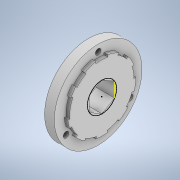
# Autodesk Inventor part: wheel_gearing_mount_short
Saved by Autodesk Inventor 2021 (Build 250183000, 183)
## iProperties
Created: 2021-01-10
Part Number: wheel_gearing_mount_short
Material: Generic
Document SubType Name: Modeling
Designer: Mateusz
Density: 1 g/cm^3
Appearance: Default
Author: Mateusz
Autodesk Inventor part; units mm, degrees
ref_plane "YZ Plane" through (0, 0, 0) normal (1, 0, 0) x (0, 1, 0)
ref_plane "XZ Plane" through (0, 0, 0) normal (0, 1, 0) x (-1, 0, 0)
ref_plane "XY Plane" through (0, 0, 0) normal (0, 0, 1) x (1, 0, 0)
sketch "Sketch1" plane through (0, 0, 0) normal (1, 0, 0) x (0, 1, 0)
  line L0 (0, 0) -> (7.5, 0)
  line L1 (7.5, 0) -> (3.75, -6.4952)
  line L2 (3.75, -6.4952) -> (-3.75, -6.4952)
  line L3 (-3.75, -6.4952) -> (-7.5, 0)
  line L4 (-7.5, 0) -> (-3.75, 6.4952)
  line L5 (-3.75, 6.4952) -> (3.75, 6.4952)
  line L6 (3.75, 6.4952) -> (7.5, 0)
  circle A0 centre (0, 0) radius 15
  dimension "d0" = 7.5
  dimension "d1" = 30
  constraints: 14 end point, 2 coincident, 1 centre point, 1 horizontal, 13 other
  measures "d0" distance of L0.start L0.end
  measures "d1" diameter of A0
extrude "Extrusion1" add sketch "Sketch1" along normal blind 10.25
sketch "Sketch2" plane through (10.25, 0, 0) normal (1, 0, 0) x (0, 0, -1)
  circle A0 centre (0, 0) radius 22.5
  line L0 (-6.4952, 3.75) -> (0, 7.5) projected
  line L1 (-6.4952, -3.75) -> (-6.4952, 3.75) projected
  line L2 (0, -7.5) -> (-6.4952, -3.75) projected
  line L3 (6.4952, -3.75) -> (0, -7.5) projected
  line L4 (6.4952, 3.75) -> (6.4952, -3.75) projected
  line L5 (0, 7.5) -> (6.4952, 3.75) projected
  dimension "d4" = 45
  constraints: 1 centre point, 1 coincident
  measures "d4" diameter of A0
extrude "Extrusion2" add sketch "Sketch2" against normal blind 5
sketch "Sketch3" plane through (10.25, 0, 0) normal (1, 0, 0) x (0, 0, -1)
  circle A0 centre (0, 19.05) radius 1.45
  circle A1 centre (-16.4978, -9.525) radius 1.45
  circle A2 centre (16.4978, -9.525) radius 1.45
  point P0 (0, 0)
  dimension "d11" = 360
  constraints: 3 centre point, 7 other
extrude "Extrusion3" cut sketch "Sketch3" against normal up to surface (5 mm away)
sketch "Sketch4" plane through (10.25, 0, 0) normal (1, 0, 0) x (0, 0, -1)
  circle A0 centre (0, 19.05) radius 1.45 projected
  line L0 (0, 19.05) -> (3, 19.05)
  line L1 (0, 19.05) -> (-3, 19.05)
  line L2 (-3, 19.05) -> (-3, 16.225)
  line L3 (3, 19.05) -> (3, 16.225)
  line L4 (-17.9978, -6.9269) -> (-15.5512, -5.5144)
  line L5 (-16.4978, -9.525) -> (-17.9978, -6.9269)
  line L6 (-16.4978, -9.525) -> (-14.9978, -12.1231)
  line L7 (-14.9978, -12.1231) -> (-12.5512, -10.7106)
  line L8 (14.9978, -12.1231) -> (12.5512, -10.7106)
  line L9 (16.4978, -9.525) -> (14.9978, -12.1231)
  line L10 (16.4978, -9.525) -> (17.9978, -6.9269)
  line L11 (17.9978, -6.9269) -> (15.5512, -5.5144)
  line L12 (12.2451, 14.5931) -> (14.5432, 12.6648)
  line L13 (14.5432, 12.6648) -> (12.7273, 10.5007)
  line L14 (12.2451, 14.5931) -> (9.947, 16.5215)
  line L15 (9.947, 16.5215) -> (8.1311, 14.3574)
  line L16 (18.7606, 3.308) -> (19.2815, 0.3536)
  line L17 (19.2815, 0.3536) -> (16.4994, -0.137)
  line L18 (18.7606, 3.308) -> (18.2396, 6.2624)
  line L19 (18.2396, 6.2624) -> (15.4575, 5.7719)
  line L20 (16.4978, -9.525) -> (14.9978, -12.1231)
  line L21 (14.9978, -12.1231) -> (12.5512, -10.7106)
  line L22 (16.4978, -9.525) -> (17.9978, -6.9269)
  line L23 (17.9978, -6.9269) -> (15.5512, -5.5144)
  arc A1 (8.7841, 15.1357) -> (3, 17.2409) centre (0, 0) ccw
  arc A2 (16.4311, -6.0224) -> (17.5, 0.0394) centre (0, 0) ccw
  arc A3 (16.4581, 5.9483) -> (13.3804, 11.279) centre (0, 0) ccw
  arc A4 (12.7273, 10.5007) -> (8.1311, 14.3574) centre (0, 0) ccw
  arc A5 (16.4994, -0.137) -> (15.4575, 5.7719) centre (0, 0) ccw
  line L24 (6.5155, -17.9011) -> (3.6964, -18.9272)
  line L25 (3.6964, -18.9272) -> (2.7302, -16.2726)
  line L26 (3.6964, -18.9272) -> (2.7302, -16.2726)
  line L27 (6.5155, -17.9011) -> (3.6964, -18.9272)
  line L28 (9.3346, -16.8751) -> (8.3683, -14.2204)
  line L29 (9.3346, -16.8751) -> (8.3683, -14.2204)
  line L30 (6.5155, -17.9011) -> (9.3346, -16.8751)
  line L31 (6.5155, -17.9011) -> (9.3346, -16.8751)
  line L32 (-6.5155, -17.9011) -> (-9.3346, -16.8751)
  line L33 (-9.3346, -16.8751) -> (-8.3683, -14.2204)
  line L34 (-9.3346, -16.8751) -> (-8.3683, -14.2204)
  line L35 (-6.5155, -17.9011) -> (-9.3346, -16.8751)
  line L36 (-3.6964, -18.9272) -> (-2.7302, -16.2726)
  line L37 (-3.6964, -18.9272) -> (-2.7302, -16.2726)
  line L38 (-6.5155, -17.9011) -> (-3.6964, -18.9272)
  line L39 (-6.5155, -17.9011) -> (-3.6964, -18.9272)
  line L40 (-16.4978, -9.525) -> (-17.9978, -6.9269)
  line L41 (-17.9978, -6.9269) -> (-15.5512, -5.5144)
  line L42 (-17.9978, -6.9269) -> (-15.5512, -5.5144)
  line L43 (-16.4978, -9.525) -> (-17.9978, -6.9269)
  line L44 (-14.9978, -12.1231) -> (-12.5512, -10.7106)
  line L45 (-14.9978, -12.1231) -> (-12.5512, -10.7106)
  line L46 (-16.4978, -9.525) -> (-14.9978, -12.1231)
  line L47 (-16.4978, -9.525) -> (-14.9978, -12.1231)
  arc A6 (8.7158, -15.1751) -> (13.4311, -11.2185) centre (0, 0) ccw
  arc A7 (-13.4311, -11.2185) -> (-8.7158, -15.1751) centre (0, 0) ccw
  arc A8 (-3.0777, -17.2272) -> (3.0777, -17.2272) centre (0, 0) ccw
  arc A9 (12.5512, -10.7106) -> (15.5512, -5.5144) centre (0, 0) ccw
  arc A10 (2.7302, -16.2726) -> (8.3683, -14.2204) centre (0, 0) ccw
  arc A11 (-8.3683, -14.2204) -> (-2.7302, -16.2726) centre (0, 0) ccw
  line L48 (-9.947, 16.5215) -> (-8.1311, 14.3574)
  line L49 (-12.2451, 14.5931) -> (-9.947, 16.5215)
  line L50 (-14.5432, 12.6648) -> (-12.7273, 10.5007)
  line L51 (-12.2451, 14.5931) -> (-14.5432, 12.6648)
  line L52 (-18.2396, 6.2624) -> (-15.4575, 5.7719)
  line L53 (-18.7606, 3.308) -> (-18.2396, 6.2624)
  line L54 (-19.2815, 0.3536) -> (-16.4994, -0.137)
  line L55 (-18.7606, 3.308) -> (-19.2815, 0.3536)
  line L56 (-17.9978, -6.9269) -> (-15.5512, -5.5144)
  line L57 (-16.4978, -9.525) -> (-17.9978, -6.9269)
  line L58 (-14.9978, -12.1231) -> (-12.5512, -10.7106)
  line L59 (-16.4978, -9.525) -> (-14.9978, -12.1231)
  line L60 (-18.7606, 3.308) -> (-17.9978, 7.7429)
  line L61 (-17.9978, 7.7429) -> (-19.5234, -1.1269)
  line L62 (-19.5234, -1.1269) -> (-16.4162, -1.6613)
  line L63 (-17.9978, 7.7429) -> (-14.8459, 7.2007)
  arc A12 (-3, 17.2409) -> (-8.7841, 15.1357) centre (0, 0) ccw
  arc A13 (-13.3804, 11.279) -> (-15.8693, 7.3768) centre (0, 0) ccw
  arc A14 (-17.4368, -1.4858) -> (-16.4311, -6.0224) centre (0, 0) ccw
  arc A15 (-15.5512, -5.5144) -> (-12.5512, -10.7106) centre (0, 0) ccw
  arc A16 (-14.8459, 7.2007) -> (-16.4162, -1.6613) centre (0, 0) ccw
  arc A17 (3, 16.225) -> (-3, 16.225) centre (0, 0) ccw
  arc A18 (-8.1311, 14.3574) -> (-12.7273, 10.5007) centre (0, 0) ccw
  line L64 (-6.4952, 3.75) -> (0, 7.5) projected
  line L65 (-6.4952, -3.75) -> (-6.4952, 3.75) projected
  line L66 (0, -7.5) -> (-6.4952, -3.75) projected
  line L67 (6.4952, -3.75) -> (0, -7.5) projected
  line L68 (6.4952, 3.75) -> (6.4952, -3.75) projected
  line L69 (0, 7.5) -> (6.4952, 3.75) projected
  point P0 (13.4311, -11.2185)
  point P1 (16.4311, -6.0224)
  point P2 (3.0777, -17.2272)
  point P3 (8.7158, -15.1751)
  point P4 (-8.7158, -15.1751)
  point P5 (-3.0777, -17.2272)
  point P6 (-16.4311, -6.0224)
  point P7 (-16.4311, -6.0224)
  point P8 (-13.4311, -11.2185)
  point P9 (-8.7158, -15.1751)
  point P10 (-3.0777, -17.2272)
  point P11 (3.0777, -17.2272)
  point P12 (8.7158, -15.1751)
  point P13 (-16.4581, 5.9483)
  point P14 (-17.5, 0.0394)
  dimension "d17" = 3
  dimension "d18" = 3
  dimension "d21" = 360
  dimension "d25" = 120
  dimension "d29" = 120
  dimension "d35" = 120
  dimension "d37" = 4.5
  dimension "d38" = 9
  constraints: 128 end point, 36 point on circle, 33 point on line, 18 centre point, 2 coincident, 2 horizontal, 2 perpendicular, 1 vertical, 169 other
  measures "d17" distance of L0.start L0.end
  measures "d18" distance of L0.start L1.end
  measures "d37" distance of L53.start L60.end
  measures "d38" distance of L60.end L61.end
extrude "Extrusion5" add sketch "Sketch4" along normal blind 1.9 contours A1 L15 A4 L13 A3 L19 A5 L17 A2 L11 A9 L8 A6 L28 A10 L25 A8 L36 A11 L33 A7 L7 A15 L4 A14 L62 A16 L63 A13 L50 A18 L48 A12 L2 A17 L3
sketch "Sketch5" plane through (12.15, 0, 0) normal (1, 0, 0) x (0, 0, -1)
  line L0 (6.4952, 3.75) -> (6.4952, -3.75) projected
  circle A0 centre (0, 0) radius 7.5
  constraints: 1 coincident, 3 other
body "Solid1"
